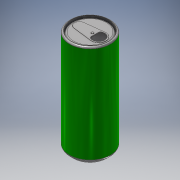
# Autodesk Inventor part: Can1
Saved by Autodesk Inventor 2016 (Build 200138000, 138)
## iProperties
Created: 2016-04-08
Part Number: Can1
Material: Stainless Steel
Document SubType Name: Modeling
Designer: Nanjar
Density: 8 g/cm^3
Appearance: Semi-Polished
Author: Nanjar
Autodesk Inventor part; units mm, degrees
ref_plane "YZ Plane" through (0, 0, 0) normal (1, 0, 0) x (0, 1, 0)
ref_plane "XZ Plane" through (0, 0, 0) normal (0, 1, 0) x (-1, 0, 0)
ref_plane "XY Plane" through (0, 0, 0) normal (0, 0, 1) x (1, 0, 0)
sketch "Sketch1" plane through (0, 0, 0) normal (0, 1, 0) x (-1, 0, 0)
  circle A0 centre (0, 0) radius 26.5
  dimension "d0" = 53
  constraints: 1 centre point, 1 coincident
  measures "d0" diameter of A0
extrude "Extrusion1" add sketch "Sketch1" along normal blind 133.2
fillet "Fillet1" radius 2 1 edges at (26.5, 133.2, 0)
chamfer "Chamfer1" distance 5.8 angle 45 1 edges at (26.5, 0, 0)
fillet "Fillet2" radius 3 1 edges at (26.5, 5.8, 0)
fillet "Fillet3" radius 2 1 edges at (20.7, 0, 0)
sketch "Sketch2" plane through (0, 0, 0) normal (0, -1, 0) x (1, 0, 0)
  circle A0 centre (0, 0) radius 19.5
  dimension "d9" = 39
  constraints: 1 centre point, 1 coincident
  measures "d9" diameter of A0
extrude "Extrusion2" cut sketch "Sketch2" against normal blind 18
fillet "Fillet4" radius 19.5 1 edges at (-19.5, 18, 0)
sketch "Sketch3" plane through (0, 133.2, 0) normal (0, 1, 0) x (1, 0, 0)
  circle A0 centre (0, 0) radius 24
  dimension "d13" = 48
  constraints: 1 centre point, 1 coincident
  measures "d13" diameter of A0
extrude "Extrusion3" cut sketch "Sketch3" against normal blind 5.5
sketch "Sketch4" plane through (0, 127.7, 0) normal (0, 1, 0) x (1, 0, 0)
  circle A0 centre (0, 0) radius 23
  dimension "d16" = 46
  constraints: 1 centre point, 1 coincident
  measures "d16" diameter of A0
extrude "Extrusion4" add sketch "Sketch4" along normal blind 4
fillet "Fillet5" radius 2 1 edges at (-23, 131.7, 0)
shell "Shell1" thickness 1 removed faces 0
sketch "Sketch5" plane through (0, 131.7, 0) normal (0, 1, 0) x (1, 0, 0)
  arc A0 (8.8312, -9.2174) -> (8.8814, 9.2297) centre (11.1313, 0) ccw
  arc A1 (-13.4595, 6.546) -> (-13.4595, -6.546) centre (-13.4595, 0) ccw
  line L0 (-13.4595, -6.546) -> (11.1882, -9.4998)
  line L1 (-13.4595, 6.546) -> (11.1313, 9.5)
  point P0 (0, 0)
  dimension "d21" = 19
  constraints: 6 point on circle, 4 end point, 2 centre point, 2 point on line
  measures "d21" diameter of A0
extrude "Extrusion5" add sketch "Sketch5" along normal blind 0.2 contours L0 A1 L1 A0
fillet "Fillet6" radius 0.2 4 edges at (-1.1356, 131.9, 8.0229) (-1.1641, 131.9, -8.023) (-20.0056, 131.9, 0) (20.6312, 131.9, -0.0285)
sketch "Sketch6" plane through (0, 131.9, 0) normal (0, 1, 0) x (1, 0, 0)
  arc A0 (11.1995, -9.2997) -> (11.1432, 9.3) centre (11.1313, 0) ccw projected
  arc A1 (6.1717, -6.1492) -> (6.1717, 6.1492) centre (11.1313, 0) ccw
  line L0 (6.1717, -6.1492) -> (6.1717, 6.1492)
  point P0 (0, 0)
  dimension "d25" = 15.8
  constraints: 2 end point, 2 point on circle, 1 centre point, 1 coincident, 1 vertical
  measures "d25" diameter of A1
extrude "Extrusion6" cut sketch "Sketch6" against normal blind 5
fillet "Fillet7" radius 3 2 edges at (6.1717, 131.3, 6.1492) (6.1717, 131.3, -6.1492)
sketch "Sketch7" plane through (0, 131.9, 0) normal (0, 1, 0) x (1, 0, 0)
  circle A0 centre (3.1307, 0) radius 1.5059
  point P0 (0, 0)
  constraints: 1 centre point
extrude "Extrusion7" add sketch "Sketch7" along normal blind 0.5
fillet "Fillet8" radius 0.2 1 edges at (1.6248, 132.4, 0)
body "Solid1"
